Autodesk Fusion 360 part; units mm, degrees
note: some values were not read from the file. Set by a fixed rule: which face or edge a step refers to.
(part 2 of 2)
sketch "Fastener Holes" plane through (103, 0, 0) normal (1, 0, 0) x (0, 1, 0)
  line L0 (72.5687, -2.0343) -> (105.8999, -2.0343)
  line L1 (105.8999, -2.0343) -> (105.243, 7.3593)
  circle A0 centre (102.5779, 2.4657) radius 1.75
  circle A1 centre (102.5779, 2.4657) radius 1.15
  circle A2 centre (51.6934, 0.4657) radius 1.15
  circle A3 centre (51.6934, 0.4657) radius 1.75
  line L2 (105.8999, -2.0343) -> (72.5687, -2.0343) construction
  line L3 (105.243, 7.3593) -> (105.8999, -2.0343) construction
  dimension "d714" = 3.5
  dimension "d716" = 4.5
  dimension "d725" = 2.3
  dimension "d794" = 2.5
  dimension "d795" = 53.9
  dimension "d796" = 3
  constraint concentric A2 A3
  constraint concentric A0 A1
  constraint equal A1 A2
  constraint equal A0 A3
  measures "d714" diameter of A0
  measures "d716" distance of L0 A0.centre
  measures "d725" diameter of A1
  measures "d794" distance of L0 A2.centre
  measures "d795" distance of A2.centre L3
  measures "d796" distance of A0.centre L3
extrude "Screw hole - 1" cut sketch "Fastener Holes" against normal up to surface (26 mm away) contours A1 | A2 bodies 2 1
extrude "Screw hole - 2" cut sketch "Fastener Holes" along normal up to surface (22 mm away) from surface at 94.25 contours A1 | A2 bodies 2 4
extrude "Insert Hole - 1" cut sketch "Fastener Holes" against normal up to surface (6 mm away) contours A0 | A1 | A2 | A3 bodies 2
extrude "Insert Hole - 2" cut sketch "Fastener Holes" along normal up to surface (4 mm away) from surface at 94.25 contours A0 | A1 | A2 | A3 bodies 2
fillet "Rouding edges" radius 0.5 8 edges at (87, 66.2544, 1.2993) (87, 74.8732, 1.6007) (87, 28.5103, -0.0204) (87, 19.8915, -0.3217) (207.25, 19.8915, -0.3217) (207.25, 28.5103, -0.0204) (207.25, 66.2544, 1.2993) (207.25, 74.8732, 1.6007) on bodies 1 2
fillet "Rouding edges" radius 1.5 2 edges at (21.75, 108.645, 5.4657) (35.25, 108.645, 5.4657) on bodies 1 2
named bodies: "Left", "Middle", "Right"
